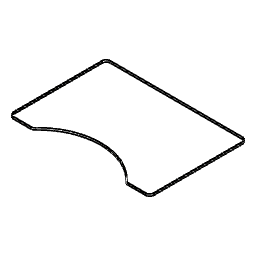
window_frame_final v4 (Autodesk Fusion 360 design; units mm, degrees)
Autodesk Fusion 360 part; units mm, degrees
sketch "Esquisse1" plane through (0, 0, 0) normal (0, 1, 0) x (1, 0, 0)
  arc A0 (305, -225) -> (325, -205) centre (305, -205) ccw
  arc A1 (-325, -205) -> (-305, -225) centre (-305, -205) ccw
  arc A2 (-223.8346, -225) -> (-209.2489, -218.6842) centre (-223.8346, -205) ccw
  line L0 (-305, -225) -> (-223.8346, -225)
  line L1 (-367.4671, -125) -> (350, -125) construction
  arc A3 (209.2489, -218.6842) -> (223.8346, -225) centre (223.8346, -205) ccw
  line L2 (325, 205) -> (325, -205)
  line L3 (-325, -205) -> (-325, 205)
  arc A4 (209.2489, -218.6842) -> (-209.2489, -218.6842) centre (0, -415) ccw
  arc A5 (-305, 225) -> (-325, 205) centre (-305, 205) ccw
  line L4 (325, 225) -> (-325, -225) construction
  line L5 (-325, 225) -> (325, -225) construction
  line L6 (-305, 225) -> (305, 225)
  arc A6 (325, 205) -> (305, 225) centre (305, 205) ccw
  line L7 (215, -225) -> (325, -225)
  line L8 (305, -225) -> (223.8346, -225)
  arc A7 (-305, 221) -> (-321, 205) centre (-305, 205) ccw
  line L9 (-321, -205) -> (-321, 205)
  arc A8 (-321, -205) -> (-305, -221) centre (-305, -205) ccw
  line L10 (-305, -221) -> (-223.8346, -221)
  arc A9 (-223.8346, -221) -> (-212.1661, -215.9474) centre (-223.8346, -205) ccw
  arc A10 (212.1661, -215.9474) -> (-212.1661, -215.9474) centre (0, -415) ccw
  arc A11 (212.1661, -215.9474) -> (223.8346, -221) centre (223.8346, -205) ccw
  line L11 (305, -221) -> (223.8346, -221)
  arc A12 (305, -221) -> (321, -205) centre (305, -205) ccw
  line L12 (321, 205) -> (321, -205)
  arc A13 (321, 205) -> (305, 221) centre (305, 205) ccw
  line L13 (-305, 221) -> (305, 221)
  line L14 (-325, -140) -> (-321, -140)
  line L15 (325, -140) -> (321, -140)
  line L16 (325, 200) -> (321, 200)
  line L17 (-325, 200) -> (-321, 200)
  line L18 (-325, 200) -> (-325, -140)
  line L19 (-321, -140) -> (-321, 200)
  line L20 (321, 200) -> (321, -140)
  line L21 (325, 200) -> (325, -140)
  line L22 (321, 200) -> (325, 200)
  line L23 (325, 200) -> (325, -140)
  line L24 (325, -140) -> (321, -140)
  line L25 (321, -140) -> (321, 200)
  line L26 (321, -140) -> (321, -205)
  line L27 (325, -140) -> (325, -205)
  line L28 (-325, -140) -> (-325, -205)
  line L29 (-321, -140) -> (-321, -205)
  point P0 (-215, -225)
  dimension "d12" = 650
  dimension "d13" = 450
  dimension "d14" = 110
  dimension "d15" = 110
  dimension "d16" = 100
  dimension "d20" = 190
  dimension "d21" = 20
  dimension "d8" = 4
  constraint horizontal L6
  constraint perpendicular L2 L6
  constraint parallel L6 L8
  constraint parallel L2 L3
  constraint coincident origin L5
  constraint coincident origin L4
  constraint coincident P0 L8
  constraint perpendicular L1 L2
  constraint perpendicular L2 L7
  constraint tangent A3 A4
  constraint tangent A3 L8
  constraint coincident L5.end L8
  constraint coincident L5.end L2
  constraint tangent A0 L8
  constraint tangent A0 L2
  constraint equal A0 A3
  constraint coincident L4.start L6
  constraint coincident L4.start L2
  constraint tangent L6 A6
  constraint tangent L2 A6
  constraint equal A3 A6
  constraint coincident L5.start L6
  constraint coincident L5.start L3
  constraint tangent A5 L6
  constraint tangent L3 A5
  constraint equal A3 A5
  constraint coincident L4.end L3
  constraint coincident L4.end L0
  constraint tangent A1 L3
  constraint tangent A1 L0
  constraint equal A1 A3
  constraint coincident P0 L0
  constraint coincident P0 A4
  constraint tangent A2 L0
  constraint tangent A2 A4
  constraint equal A2 A3
  constraint coincident L3 L14.start
  constraint coincident L9 L14.end
  constraint perpendicular L9 L14
  constraint coincident L2 L15.start
  constraint coincident L12 L15.end
  constraint perpendicular L12 L15
  constraint coincident L2 L16.start
  constraint coincident L12 L16.end
  constraint perpendicular L12 L16
  constraint coincident L3 L17.start
  constraint coincident L9 L17.end
  constraint perpendicular L9 L17
  measures "d12" distance of L4.start L5.start
  measures "d13" distance of L4.end L5.start
  measures "d14" distance of P0 L3
  measures "d15" distance of L7.start L2
  measures "d16" distance of L1 L8
  measures "d20" distance of A4.centre L8
  measures "d21" radius of A3
extrude "Extrusion1" add sketch "Esquisse1" along normal blind 9 contours A0 A1 A2 L0 A3 L2 L3 A4 L7 L8 L9 A8 L10 A9 A10 A11 L11 A12 L12 L14 L15 L24 L26 L27 L28 L29 | L2 L12 L15 L16 L20 L21 L22 L23 L24 L25 | L2 L3 A5 L6 A6 A7 L9 L12 A13 L13 L16 L17 L22 | L3 L9 L14 L17 L18 L19
